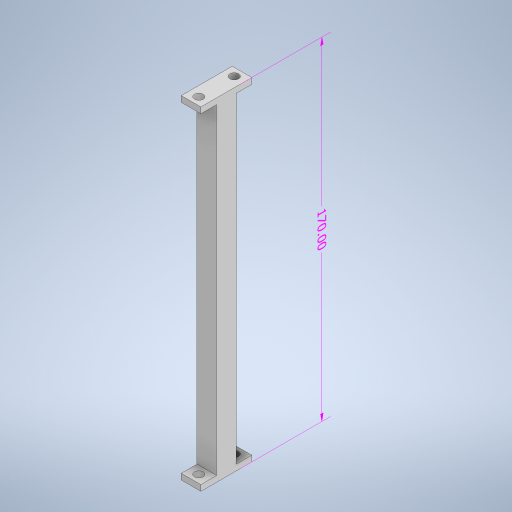
# Autodesk Inventor part: basket_pilar
Saved by Autodesk Inventor 2024 (Build 280153000, 153)
## iProperties
Created: 2024-05-18
Part Number: basket_pilar
Material: Generic
Document SubType Name: Modeling
Designer: inigo
Density: 1 g/cm^3
Appearance: Default
Author: inigo
Autodesk Inventor part; units mm, degrees
ref_plane "YZ Plane" through (0, 0, 0) normal (1, 0, 0) x (0, 1, 0)
ref_plane "XZ Plane" through (0, 0, 0) normal (0, 1, 0) x (-1, 0, 0)
ref_plane "XY Plane" through (0, 0, 0) normal (0, 0, 1) x (1, 0, 0)
sketch "Sketch1" plane through (0, 0, 0) normal (0, 1, 0) x (-1, 0, 0)
  line L0 (5, 5) -> (-5, 5)
  line L1 (-5, 5) -> (-5, -5)
  line L2 (-5, -5) -> (5, -5)
  line L3 (5, -5) -> (5, 5)
  line L4 (5, 5) -> (-5, -5) construction
  line L5 (-5, 5) -> (5, -5) construction
  circle A0 centre (0, 9) radius 2.25
  line L6 (5, 0) -> (7.8618, 0)
  circle A1 centre (0, -9) radius 2.25
  line L7 (5, -9) -> (5, -5)
  line L8 (-5, -9) -> (-5, -5)
  line L9 (-5, 5) -> (5, 5)
  line L10 (5, 5) -> (5, 13)
  line L11 (5, 13) -> (-5, 13)
  line L12 (-5, 13) -> (-5, 5)
  line L13 (-5, -5) -> (5, -5)
  line L14 (5, -5) -> (5, -13)
  line L15 (5, -13) -> (-5, -13)
  line L16 (-5, -13) -> (-5, -5)
  point P0 (0, 0)
  dimension "d0" = 10
  dimension "d1" = 10
  dimension "d2" = 4.5
  dimension "d4" = 4
  dimension "d17" = 4
  constraints: 34 end point, 6 symmetric about line, 4 parallel, 3 horizontal, 3 midpoint, 2 centre point, 2 perpendicular, 1 other
  measures "d0" distance of L2.end L1.end
  measures "d1" distance of L1.end L0.end
  measures "d2" diameter of A0
  measures "d4" distance from line of L0 A0.centre
  measures "d17" distance from line of L11 A0.centre
extrude "Extrusion1" add sketch "Sketch1" along normal blind 3
sketch "Sketch2" plane through (0, 3, 0) normal (0, 1, 0) x (1, 0, 0)
  line L0 (-5, 5) -> (-5, -5) projected
  line L1 (5, -5) -> (-5, -5)
  line L2 (-5, -5) -> (-5, 5)
  line L3 (-5, 5) -> (5, 5)
  line L4 (5, 5) -> (5, -5)
  line L5 (5, -5) -> (-5, 5) construction
  line L6 (-5, -5) -> (5, 5) construction
  point P0 (0, 0)
  point P1 (-5, 9)
  point P2 (-5, -9)
  dimension "d8" = 10
  constraints: 13 end point, 2 midpoint, 2 parallel, 1 horizontal, 1 perpendicular
  measures "d8" distance of L0.end L0.start
extrude "Extrusion2" add sketch "Sketch2" along normal blind 82
mirror "Mirror1" about plane through (0, 85, 0) normal (0, 1, 0) of "Extrusion1", "Extrusion2"
body "Solid1"
